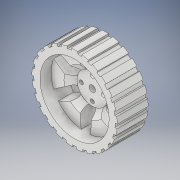
# Autodesk Inventor part: Wheel2
Saved by Autodesk Inventor 2017 (Build 210142000, 142)
## iProperties
Created: 2018-02-27
Part Number: Wheel2
Material: PAEK Plastic
Document SubType Name: Modeling
Designer: bradl
Density: 1.32 g/cm^3
Appearance: Smooth - White
Author: bradl
Autodesk Inventor part; units mm, degrees
ref_plane "YZ Plane" through (0, 0, 0) normal (1, 0, 0) x (0, 1, 0)
ref_plane "XZ Plane" through (0, 0, 0) normal (0, 1, 0) x (-1, 0, 0)
ref_plane "XY Plane" through (0, 0, 0) normal (0, 0, 1) x (1, 0, 0)
sketch "Sketch1" plane through (0, 0, 0) normal (0, 0, 1) x (1, 0, 0)
  circle A0 centre (0, 0) radius 2
  circle A1 centre (0, 6.858) radius 1.27
  circle A2 centre (6.858, 0) radius 1.27
  circle A3 centre (0, -6.858) radius 1.27
  circle A4 centre (-6.858, 0) radius 1.27
  line L0 (-2, 25.3211) -> (-2, 26.5911)
  line L1 (-2, 26.5911) -> (2, 26.5911)
  line L2 (2, 26.5911) -> (2, 25.3211)
  line L3 (-8.5501, 25.2583) -> (-4.6758, 26.2531)
  line L4 (-4.6758, 26.2531) -> (-4.3599, 25.023)
  line L5 (-8.2343, 24.0282) -> (-8.5501, 25.2583)
  line L6 (-14.563, 22.3385) -> (-11.0578, 24.2655)
  line L7 (-11.0578, 24.2655) -> (-10.4459, 23.1526)
  line L8 (-13.9512, 21.2256) -> (-14.563, 22.3385)
  line L9 (-19.6608, 18.015) -> (-16.7449, 20.7532)
  line L10 (-16.7449, 20.7532) -> (-15.8756, 19.8274)
  line L11 (-18.7914, 17.0892) -> (-19.6608, 18.015)
  line L12 (-23.5233, 12.5596) -> (-21.38, 15.9369)
  line L13 (-21.38, 15.9369) -> (-20.3077, 15.2564)
  line L14 (-22.451, 11.8791) -> (-23.5233, 12.5596)
  line L15 (-25.9077, 6.315) -> (-24.6716, 10.1192)
  line L16 (-24.6716, 10.1192) -> (-23.4638, 9.7268)
  line L17 (-24.6999, 5.9225) -> (-25.9077, 6.315)
  line L18 (-26.6642, -0.3264) -> (-26.4131, 3.6657)
  line L19 (-26.4131, 3.6657) -> (-25.1456, 3.586)
  line L20 (-25.3968, -0.4061) -> (-26.6642, -0.3264)
  line L21 (-25.7454, -6.9473) -> (-26.4949, -3.0181)
  line L22 (-26.4949, -3.0181) -> (-25.2474, -2.7801)
  line L23 (-24.4979, -6.7093) -> (-25.7454, -6.9473)
  line L24 (-23.2088, -13.1316) -> (-24.9119, -9.5123)
  line L25 (-24.9119, -9.5123) -> (-23.7628, -8.9716)
  line L26 (-22.0597, -12.5909) -> (-23.2088, -13.1316)
  line L27 (-19.214, -18.4909) -> (-21.7637, -15.4088)
  line L28 (-21.7637, -15.4088) -> (-20.7851, -14.5993)
  line L29 (-18.2354, -17.6813) -> (-19.214, -18.4909)
  line L30 (-14.0118, -22.6883) -> (-17.2479, -20.3371)
  line L31 (-17.2479, -20.3371) -> (-16.5014, -19.3097)
  line L32 (-13.2654, -21.6608) -> (-14.0118, -22.6883)
  line L33 (-7.9293, -25.4601) -> (-11.6484, -23.9876)
  line L34 (-11.6484, -23.9876) -> (-11.1809, -22.8067)
  line L35 (-7.4618, -24.2792) -> (-7.9293, -25.4601)
  line L36 (-1.3485, -26.6321) -> (-5.317, -26.1308)
  line L37 (-5.317, -26.1308) -> (-5.1578, -24.8708)
  line L38 (-1.1894, -25.3721) -> (-1.3485, -26.6321)
  line L39 (5.317, -26.1308) -> (1.3485, -26.6321)
  line L40 (1.3485, -26.6321) -> (1.1894, -25.3721)
  line L41 (5.1578, -24.8708) -> (5.317, -26.1308)
  line L42 (11.6484, -23.9876) -> (7.9293, -25.4601)
  line L43 (7.9293, -25.4601) -> (7.4618, -24.2792)
  line L44 (11.1809, -22.8067) -> (11.6484, -23.9876)
  line L45 (17.2479, -20.3371) -> (14.0118, -22.6883)
  line L46 (14.0118, -22.6883) -> (13.2654, -21.6608)
  line L47 (16.5014, -19.3097) -> (17.2479, -20.3371)
  line L48 (21.7637, -15.4088) -> (19.214, -18.4909)
  line L49 (19.214, -18.4909) -> (18.2354, -17.6813)
  line L50 (20.7851, -14.5993) -> (21.7637, -15.4088)
  line L51 (24.9119, -9.5123) -> (23.2088, -13.1316)
  line L52 (23.2088, -13.1316) -> (22.0597, -12.5909)
  line L53 (23.7628, -8.9716) -> (24.9119, -9.5123)
  line L54 (26.4949, -3.0181) -> (25.7454, -6.9473)
  line L55 (25.7454, -6.9473) -> (24.4979, -6.7093)
  line L56 (25.2474, -2.7801) -> (26.4949, -3.0181)
  line L57 (26.4131, 3.6657) -> (26.6642, -0.3264)
  line L58 (26.6642, -0.3264) -> (25.3968, -0.4061)
  line L59 (25.1456, 3.586) -> (26.4131, 3.6657)
  line L60 (24.6716, 10.1192) -> (25.9077, 6.315)
  line L61 (25.9077, 6.315) -> (24.6999, 5.9225)
  line L62 (23.4638, 9.7268) -> (24.6716, 10.1192)
  line L63 (21.38, 15.9369) -> (23.5233, 12.5596)
  line L64 (23.5233, 12.5596) -> (22.451, 11.8791)
  line L65 (20.3077, 15.2564) -> (21.38, 15.9369)
  line L66 (16.7449, 20.7532) -> (19.6608, 18.015)
  line L67 (19.6608, 18.015) -> (18.7914, 17.0892)
  line L68 (15.8756, 19.8274) -> (16.7449, 20.7532)
  line L69 (11.0578, 24.2655) -> (14.563, 22.3385)
  line L70 (14.563, 22.3385) -> (13.9512, 21.2256)
  line L71 (10.4459, 23.1526) -> (11.0578, 24.2655)
  line L72 (4.6758, 26.2531) -> (8.5501, 25.2583)
  line L73 (8.5501, 25.2583) -> (8.2343, 24.0282)
  line L74 (4.3599, 25.023) -> (4.6758, 26.2531)
  arc A5 (4.3599, 25.023) -> (2, 25.3211) centre (0, 0) ccw
  arc A6 (10.4459, 23.1526) -> (8.2343, 24.0282) centre (0, 0) ccw
  arc A7 (-2, 25.3211) -> (-4.3599, 25.023) centre (0, 0) ccw
  arc A8 (-8.2343, 24.0282) -> (-10.4459, 23.1526) centre (0, 0) ccw
  arc A9 (-13.9512, 21.2256) -> (-15.8756, 19.8274) centre (0, 0) ccw
  arc A10 (-18.7914, 17.0892) -> (-20.3077, 15.2564) centre (0, 0) ccw
  arc A11 (-22.451, 11.8791) -> (-23.4638, 9.7268) centre (0, 0) ccw
  arc A12 (-24.6999, 5.9225) -> (-25.1456, 3.586) centre (0, 0) ccw
  arc A13 (-25.3968, -0.4061) -> (-25.2474, -2.7801) centre (0, 0) ccw
  arc A14 (-24.4979, -6.7093) -> (-23.7628, -8.9716) centre (0, 0) ccw
  arc A15 (-22.0597, -12.5909) -> (-20.7851, -14.5993) centre (0, 0) ccw
  arc A16 (-18.2354, -17.6813) -> (-16.5014, -19.3097) centre (0, 0) ccw
  arc A17 (-13.2654, -21.6608) -> (-11.1809, -22.8067) centre (0, 0) ccw
  arc A18 (-7.4618, -24.2792) -> (-5.1578, -24.8708) centre (0, 0) ccw
  arc A19 (-1.1894, -25.3721) -> (1.1894, -25.3721) centre (0, 0) ccw
  arc A20 (5.1578, -24.8708) -> (7.4618, -24.2792) centre (0, 0) ccw
  arc A21 (11.1809, -22.8067) -> (13.2654, -21.6608) centre (0, 0) ccw
  arc A22 (16.5014, -19.3097) -> (18.2354, -17.6813) centre (0, 0) ccw
  arc A23 (20.7851, -14.5993) -> (22.0597, -12.5909) centre (0, 0) ccw
  arc A24 (23.7628, -8.9716) -> (24.4979, -6.7093) centre (0, 0) ccw
  arc A25 (25.2474, -2.7801) -> (25.3968, -0.4061) centre (0, 0) ccw
  arc A26 (25.1456, 3.586) -> (24.6999, 5.9225) centre (0, 0) ccw
  arc A27 (23.4638, 9.7268) -> (22.451, 11.8791) centre (0, 0) ccw
  arc A28 (20.3077, 15.2564) -> (18.7914, 17.0892) centre (0, 0) ccw
  arc A29 (15.8756, 19.8274) -> (13.9512, 21.2256) centre (0, 0) ccw
  circle A30 centre (0, 0) radius 2
  circle A31 centre (6.858, 0) radius 1.27
  circle A32 centre (0, -6.858) radius 1.27
  circle A33 centre (0, 6.858) radius 1.27
  circle A34 centre (-6.858, 0) radius 1.27
  dimension "d2" = 1.27
  dimension "d3" = 360
  constraints: 150 end point, 50 point on circle, 35 centre point, 6 coincident, 5 concentric, 2 tangent, 1 perpendicular, 1 vertical, 176 other
  measures "d2" distance of L0.start L0.end
extrude "Extrusion1" add sketch "Sketch1" along normal blind 19.304
sketch "Sketch2" plane through (0, 0, 19.304) normal (0, 0, 1) x (1, 0, 0)
  circle A0 centre (0, 0) radius 21.59
  circle A1 centre (-6.858, 0) radius 1.27 projected
  circle A2 centre (0, 0) radius 2 projected
  circle A3 centre (0, 6.858) radius 1.27 projected
  circle A4 centre (6.858, 0) radius 1.27 projected
  circle A5 centre (0, -6.858) radius 1.27 projected
  circle A6 centre (0, 0) radius 2 projected
  circle A7 centre (0, 0) radius 2
  circle A8 centre (0, 6.858) radius 1.27
  circle A9 centre (-6.858, 0) radius 1.27
  circle A10 centre (0, -6.858) radius 1.27 projected
  circle A11 centre (0, -6.858) radius 1.27
  circle A12 centre (6.858, 0) radius 1.27
  circle A13 centre (0, 0) radius 9.525
  dimension "d6" = 43.18
  dimension "d7" = 19.05
  constraints: 7 centre point, 7 coincident, 3 concentric
  measures "d6" diameter of A0
  measures "d7" diameter of A13
extrude "Extrusion2" cut sketch "Sketch2" against normal blind 16.51 contours A0
sketch "Sketch3" plane through (0, 0, 2.794) normal (0, 0, 1) x (1, 0, 0)
  circle A0 centre (0, 0) radius 9.525 projected
  circle A1 centre (0, 0) radius 21.59 projected
  line L0 (0, 0) -> (0, 21.59) construction
  line L1 (0, 0) -> (-8.2621, 19.9466) construction
  line L2 (0, 0) -> (-15.2664, 15.2664) construction
  line L3 (0, 0) -> (-19.9466, 8.2621) construction
  line L4 (0, 0) -> (-21.59, 0) construction
  line L5 (0, 0) -> (-19.9466, -8.2621) construction
  line L6 (0, 0) -> (-15.2664, -15.2664) construction
  line L7 (0, 0) -> (-8.2621, -19.9466) construction
  line L8 (0, 0) -> (0, -21.59) construction
  line L9 (0, 0) -> (8.2621, -19.9466) construction
  line L10 (0, 0) -> (15.2664, -15.2664) construction
  line L11 (0, 0) -> (19.9466, -8.2621) construction
  line L12 (0, 0) -> (21.59, 0) construction
  line L13 (0, 0) -> (19.9466, 8.2621) construction
  line L14 (0, 0) -> (15.2664, 15.2664) construction
  line L15 (0, 0) -> (8.2621, 19.9466) construction
  arc A2 (-9.0144, -3.0769) -> (-9.525, 0) centre (0, 0) ccw
  line L16 (-8.8, -3.6451) -> (-9.525, 0) construction
  line L17 (-9.525, 0) -> (-19.9466, -8.2621) construction
  spline S0 degree 2 poles (-8.8, -3.6451) (-9.525, 0) (-19.9466, -8.2621) knots 1 1 1 2 2 2
  line L18 (-8.8, 3.6451) -> (-9.525, 0) construction
  line L19 (-9.525, 0) -> (-19.9466, 8.2621) construction
  spline S1 degree 2 poles (-8.8, 3.6451) (-9.525, 0) (-19.9466, 8.2621) knots 1 1 1 2 2 2
  spline S2 degree 2 poles (-3.6451, -8.8) (0, -9.525) (-8.2621, -19.9466) knots 1 1 1 2 2 2
  line L20 (-3.6451, -8.8) -> (0, -9.525) construction
  line L21 (0, -9.525) -> (-8.2621, -19.9466) construction
  spline S3 degree 2 poles (3.6451, -8.8) (0, -9.525) (8.2621, -19.9466) knots 1 1 1 2 2 2
  line L22 (3.6451, -8.8) -> (0, -9.525) construction
  line L23 (0, -9.525) -> (8.2621, -19.9466) construction
  spline S4 degree 2 poles (8.8, -3.6451) (9.525, 0) (19.9466, -8.2621) knots 1 1 1 2 2 2
  line L24 (8.8, -3.6451) -> (9.525, 0) construction
  line L25 (9.525, 0) -> (19.9466, -8.2621) construction
  spline S5 degree 2 poles (8.8, 3.6451) (9.525, 0) (19.9466, 8.2621) knots 1 1 1 2 2 2
  line L26 (8.8, 3.6451) -> (9.525, 0) construction
  line L27 (9.525, 0) -> (19.9466, 8.2621) construction
  spline S6 degree 2 poles (3.6451, 8.8) (0, 9.525) (8.2621, 19.9466) knots 1 1 1 2 2 2
  line L28 (3.6451, 8.8) -> (0, 9.525) construction
  line L29 (0, 9.525) -> (8.2621, 19.9466) construction
  spline S7 degree 2 poles (-3.6451, 8.8) (0, 9.525) (-8.2621, 19.9466) knots 1 1 1 2 2 2
  line L30 (-3.6451, 8.8) -> (0, 9.525) construction
  line L31 (0, 9.525) -> (-8.2621, 19.9466) construction
  arc A3 (-8.2621, -19.9466) -> (8.2621, -19.9466) centre (0, 0) ccw
  arc A4 (19.9466, -8.2621) -> (19.9466, 8.2621) centre (0, 0) ccw
  arc A5 (8.2621, 19.9466) -> (-8.2621, 19.9466) centre (0, 0) ccw
  arc A6 (-19.9466, 8.2621) -> (-19.9466, -8.2621) centre (0, 0) ccw
  dimension "d12" = 360
  dimension "d16" = 360
  constraints: 32 end point, 12 point on circle, 5 centre point, 5 coincident, 3 point on line, 1 concentric, 1 vertical, 1 vertical alignment, 124 other
extrude "Extrusion3" add sketch "Sketch3" along normal blind 9.525 contours S5 A0 S4 S3 S2 S0 S1 S7 S6 | A0 S5 | S6 A0 | S7 A0 | A0 S4 | S1 A0 S0 A1 | A0 S3 | A0 S2
pattern_circular "Circular Pattern1" count 6 over 360 about axis through (0, 0, 0) along (0, 0, 1) of "Extrusion3"
sketch "Sketch4" plane through (0, 0, 19.304) normal (0, 0, 1) x (1, 0, 0)
  circle A0 centre (0, 0) radius 9.525 projected
  circle A1 centre (0, 0) radius 2 projected
  circle A2 centre (-6.858, 0) radius 1.27 projected
  circle A3 centre (0, -6.858) radius 1.27 projected
  circle A4 centre (6.858, 0) radius 1.27 projected
  circle A5 centre (0, 6.858) radius 1.27 projected
  circle A6 centre (0, 0) radius 2
  circle A7 centre (0, 6.858) radius 1.27
  circle A8 centre (6.858, 0) radius 1.27
  circle A9 centre (0, -6.858) radius 1.27
  circle A10 centre (-6.858, 0) radius 1.27
  constraints: 5 centre point, 5 coincident, 4 concentric
extrude "Extrusion4" cut sketch "Sketch4" against normal blind 52.3875 contours A1 | A2 | A3 | A4 | A5
sketch "Sketch5" plane through (0, 0, 19.304) normal (0, 0, 1) x (1, 0, 0)
  circle A0 centre (0, 0) radius 9.525
  constraints: 1 centre point, 1 coincident
extrude "Extrusion5" cut sketch "Sketch5" against normal blind 11.1125
chamfer "Chamfer1" distance 4.064 angle 45 6 edges at (-9.525, 0, 12.319) (-4.7625, 8.2489, 12.319) (4.7625, 8.2489, 12.319) (9.525, 0, 12.319) (4.7625, -8.2489, 12.319) (-4.7625, -8.2489, 12.319)
body "Solid1"
